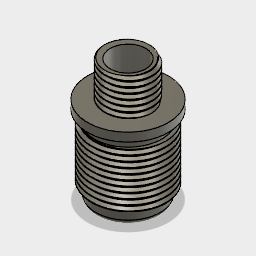
adopter(base) v4 (Autodesk Fusion 360 design; units mm, degrees)
Autodesk Fusion 360 part; units mm, degrees
sketch "スケッチ1" plane through (0, 0, 0) normal (0, 1, 0) x (1, 0, 0)
  circle A0 centre (0, 0) radius 4.5
  constraint coincident A0.centre origin
extrude "押し出し1" add sketch "スケッチ1" along normal blind 6.5
sketch "スケッチ2" plane through (0, 0, 0) normal (0, -1, 0) x (1, 0, 0)
  circle A0 centre (0, 0) radius 4.5
  circle A1 centre (0, 0) radius 7.5
  constraint concentric A0 A1
extrude "押し出し2" add sketch "スケッチ2" along normal blind 1.6 contours A0 | A1
thread "ねじ1" "ISO Metric profile 9.0 M9x1 6g" major diameter 8.884 minor diameter 7.744 pitch 1 angle 60 modelled left hand crest width 0.125 on face at (4.4776, 4.3333, 0.4481) crest through (4.442, -0.0625, 0)
sketch "スケッチ3" plane through (0, 0, 0) normal (1, 0, 0) x (0, 0, -1)
sketch "スケッチ4" plane through (0, -1.6, 0) normal (0, -1, 0) x (1, 0, 0)
  circle A0 centre (0, 0) radius 7.5
  circle A1 centre (0, 0) radius 7
  constraint concentric A0 A1
sketch "スケッチ5" plane through (0, -1.6, 0) normal (0, -1, 0) x (1, 0, 0)
  circle A0 centre (0, 0) radius 7.5
  circle A1 centre (0, 0) radius 6.25
  dimension "d7" = 12.5
  constraint concentric A0 A1
  measures "d7" diameter of A1
extrude "押し出し4" add sketch "スケッチ5" along normal blind 1.7 contours A1
sketch "スケッチ6" plane through (0, -3.3, 0) normal (0, -1, 0) x (1, 0, 0)
  circle A0 centre (0, 0) radius 6.25
  circle A1 centre (0, 0) radius 7
  constraint concentric A0 A1
extrude "押し出し5" add sketch "スケッチ6" along normal blind 10 contours A0 | A1
sketch "スケッチ7" plane through (0, -13.3, 0) normal (0, -1, 0) x (1, 0, 0)
  circle A0 centre (0, 0) radius 7
  circle A1 centre (0, 0) radius 6
  constraint concentric A0 A1
extrude "押し出し6" add sketch "スケッチ7" along normal blind 2.8 contours A1
thread "ねじ3" "ISO Metric profile 14.0 M14x1 6g" major diameter 13.884 minor diameter 12.741 pitch 1 angle 60 modelled left hand crest width 0.125 on face at (6.9913, -9.9667, -0.3489) crest through (6.942, -3.2375, 0)
fillet "フィレット1" radius 0.9 1 edges at (-5.594, -16.1, -2.1697)
sketch "スケッチ8" plane through (0, 6.5, 0) normal (0, 1, 0) x (-1, 0, 0)
  spline S0 degree 3 poles (-3.712, -1.1015) (-3.6021, -1.5992) (-3.3948, -2.0703) (-2.8054, -2.9194) (-2.4247, -3.2863) (-1.5336, -3.8633) (-1.0291, -4.0634) (0.0417, -4.2642) (0.5985, -4.2576) (1.5062, -4.0698) (1.8618, -3.946) (2.5382, -3.6077) (2.8552, -3.3933) (3.141, -3.141) knots 0 0 0 0 0.152913 0.152913 0.309919 0.309919 0.471015 0.471015 0.6362 0.6362 0.748448 0.748448 0.862517 0.862517 0.862517 0.862517
  arc A0 (3.141, -3.141) -> (4.442, 0) centre (0, 0) ccw
  spline S1 degree 3 poles (4.442, 0) (4.4067, 0.5695) (4.2617, 1.1267) (3.7701, 2.1407) (3.4329, 2.5899) (2.6139, 3.3227) (2.1435, 3.6031) (1.1339, 3.9608) (0.6062, 4.0395) (-0.265, 3.9968) (-0.6048, 3.9358) (-1.2541, 3.7289) (-1.5613, 3.5853) (-1.8459, 3.4037) knots 0 0 0 0 0.17117 0.17117 0.338243 0.338243 0.501216 0.501216 0.660089 0.660089 0.76346 0.76346 0.865009 0.865009 0.865009 0.865009
  arc A1 (-1.8459, 3.4037) -> (-3.712, -1.1015) centre (0, 0) ccw
  circle A2 centre (0, 0) radius 3.3
  dimension "d17" = 6.6
  constraint concentric A0 A2
  measures "d17" diameter of A2
extrude "押し出し7" cut sketch "スケッチ8" against normal blind 23 contours A2
extrude "押し出し3" [suppressed]
thread "ねじ2" [suppressed]
delete_face "面を削除1" [suppressed]
